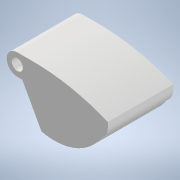
# Autodesk Inventor part: Dedo_4
Saved by Autodesk Inventor 2020 (Build 240168000, 168)
## iProperties
Created: 2021-07-29
Part Number: Dedo_4
Material: Generic
Document SubType Name: Modeling
Designer: chalo
Density: 1 g/cm^3
Appearance: Default
Author: chalo
Autodesk Inventor part; units mm, degrees
ref_plane "YZ Plane" through (0, 0, 0) normal (1, 0, 0) x (0, 1, 0)
ref_plane "XZ Plane" through (0, 0, 0) normal (0, 1, 0) x (-1, 0, 0)
ref_plane "XY Plane" through (0, 0, 0) normal (0, 0, 1) x (1, 0, 0)
sketch "Sketch1" plane through (0, 0, 0) normal (0, 0, 1) x (1, 0, 0)
  line L0 (-3.3, -2.1) -> (-0.3, -2.1) projected
  arc A0 (-0.3, -2.1) -> (-0.3, 2.1) centre (-0.3, 0) ccw projected
  line L1 (-0.3, 2.1) -> (-3.8, 2.1) projected
  line L2 (-3.8, 2.1) -> (-3.8, 0.6) projected
  line L3 (-3.3, 0.6) -> (-3.8, 0.6) projected
  line L4 (-3.3, -2.1) -> (-3.3, 0.6) projected
  circle A1 centre (-0.3, 0) radius 1.1 projected
  circle A2 centre (-0.3, 0) radius 2.1
  point P0 (0, 0)
  point P1 (-0.3, 2.1)
  constraints: 1 centre point, 1 coincident, 1 concentric
extrude "Extrusion1" add sketch "Sketch1" along normal blind 13 contours A2 A0
sketch "Sketch2" plane through (-0.3, 0, 13) normal (0, 0, 1) x (1, 0, 0)
  circle A0 centre (0, 0) radius 2.1 projected
  circle A1 centre (0, 0) radius 1.1 projected
  circle A2 centre (0, 0) radius 2.1 projected
  line L0 (0, 2.1) -> (3, 2.1)
  circle A3 centre (0, 0) radius 2.1 projected
  line L1 (0, -2.1) -> (1, -2.1)
  arc A4 (18, -0.9) -> (3, 2.1) centre (3, -36.9) ccw
  line L2 (18, -0.9) -> (18, -1.9)
  arc A5 (16.8, -4.1) -> (18, -1.9) centre (15.3833, -1.9) ccw
  arc A6 (4.8, -9.1) -> (16.8, -4.1) centre (7.3869, 1.5915) ccw
  line L3 (4.8, -9.1) -> (1, -2.1)
  point P0 (0.3, 0)
  dimension "d2" = 3
  dimension "d3" = 1
  dimension "d4" = 15
  dimension "d5" = 3
  dimension "d6" = 1
  dimension "d7" = 1.2
  dimension "d8" = 2.2
  dimension "d9" = 12
  dimension "d10" = 5
  dimension "d11" = 11
  constraints: 8 end point, 7 point on circle, 5 tangent, 4 horizontal, 3 centre point, 1 vertical, 1 vertical alignment, 1 other
  measures "d2" distance of L0.start L0.end
  measures "d3" distance of L1.start L1.end
  measures "d4" horizontal distance of L2.start L0.end
  measures "d5" vertical distance of L0.end L2.start
  measures "d6" distance of L2.start L2.end
  measures "d7" distance from line of L2 A5.start
  measures "d8" vertical distance of L2.end A5.start
  measures "d9" horizontal distance of L3.start A5.start
  measures "d10" vertical distance of A5.start L3.start
  measures "d11" radius of A6
extrude "Extrusion2" add sketch "Sketch2" against normal blind 13 contours A0 L0 A4 L2 A5 A6 L3 L1
ref_plane "Work Plane1" through (-0.3, 0, 6.5) normal (0, 0, -1) x (-1, 0, 0)
sketch "Sketch3" plane through (-0.3, 0, 6.5) normal (0, 0, -1) x (-1, 0, 0)
  arc A0 (0, -2.1) -> (0, 2.1) centre (0, 0) ccw projected
  line L0 (0, 2.1) -> (-3, 2.1) projected
  arc A1 (-3, 2.1) -> (-18, -0.9) centre (-3, -36.9) ccw projected
  line L1 (-18, -0.9) -> (-18, -1.9) projected
  arc A2 (-18, -1.9) -> (-16.8, -4.1) centre (-15.3833, -1.9) ccw projected
  arc A3 (-16.8, -4.1) -> (-4.8, -9.1) centre (-7.3869, 1.5915) ccw projected
  line L2 (-4.8, -9.1) -> (-1, -2.1) projected
  line L3 (-1, -2.1) -> (0, -2.1) projected
  circle A4 centre (0, 0) radius 1.1 projected
  arc A5 (-16.8, -4.1) -> (-4.8, -9.1) centre (-7.3869, 1.5915) ccw projected
  line L4 (-4.8, -9.1) -> (9.3272, -1.5885)
  line L5 (-4.8, -9.1) -> (-1, -2.1) projected
  line L6 (-3.0714, -5.9158) -> (8.3882, 0.1774)
  line L7 (-4.8, -9.1) -> (0.2, -9.1) construction
  line L8 (8.3882, 0.1774) -> (9.3272, -1.5885)
  circle A6 centre (8.8577, -0.7055) radius 1.1
  point P0 (-0.3, 0)
  point P1 (7.9836, -0.0377)
  point P2 (-3.0714, -5.9158)
  point P3 (8.9225, -1.8036)
  dimension "d14" = 5
  dimension "d15" = 28
  dimension "d16" = 2
  dimension "d17" = 2.2
  dimension "d18" = 16
  constraints: 8 end point, 1 centre point, 1 horizontal, 1 midpoint, 1 parallel, 1 perpendicular, 1 point on line
  measures "d14" distance of L2.start L7.end
  measures "d15" angle of L7 L4
  measures "d16" distance from line of L6 L2.start
  measures "d17" diameter of A6
  measures "d18" distance of L2.start L4.end
extrude "Extrusion3" add sketch "Sketch3" along normal mid plane 3 contours L6 A6 L4 L2 | A6 L4 L8 L6 | L6 L8 L4 A6
sketch "Sketch4" plane through (-0.3, 0, 5) normal (0, 0, -1) x (-1, 0, 0)
  arc A0 (8.9225, -1.8036) -> (7.9836, -0.0377) centre (8.8577, -0.7055) ccw projected
  line L0 (7.9836, -0.0377) -> (-3.0714, -5.9158) projected
  line L1 (-4.8, -9.1) -> (-3.0714, -5.9158) projected
  line L2 (-4.8, -9.1) -> (8.9225, -1.8036) projected
  circle A1 centre (8.8577, -0.7055) radius 2
  circle A2 centre (8.8577, -0.7055) radius 1.1
  point P0 (-0.3, 0)
  point P1 (6.8589, -0.6357)
  point P2 (7.7979, -2.4016)
  dimension "d21" = 4
  constraints: 2 centre point, 2 coincident, 1 concentric
  measures "d21" diameter of A1
extrude "Extrusion4" add sketch "Sketch4" against normal blind 3 contours A0 L0 A1 L2
sketch "Sketch5" plane through (-0.3, 0, 5) normal (0, 0, -1) x (-1, 0, 0)
  arc A0 (7.7979, -2.4016) -> (6.8589, -0.6357) centre (8.8577, -0.7055) ccw projected
  line L0 (6.8589, -0.6357) -> (-3.0714, -5.9158) projected
  line L1 (-4.8, -9.1) -> (-3.0714, -5.9158) projected
  line L2 (-4.8, -9.1) -> (7.7979, -2.4016) projected
  circle A1 centre (8.8577, -0.7055) radius 1.1
  point P0 (-0.3, 0)
  dimension "d24" = 2.2
  constraints: 1 centre point, 1 coincident
  measures "d24" diameter of A1
extrude "Extrusion5" cut sketch "Sketch5" against normal blind 3 contours A1
body "Solid1"
